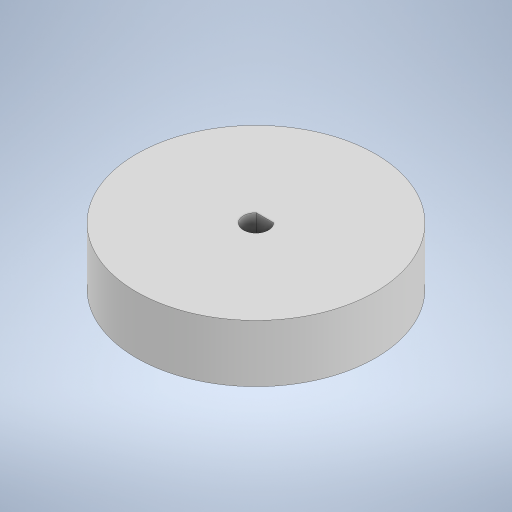
# Autodesk Inventor part: motor_gearMK2
Saved by Autodesk Inventor 2023 (Build 270158000, 158)
## iProperties
Created: 2023-03-07
Part Number: motor_gearMK2
Material: Generic
Document SubType Name: Modeling
Designer: caleb
Density: 1 g/cm^3
Appearance: Default
Author: caleb
Autodesk Inventor part; units mm, degrees
ref_plane "YZ Plane" through (0, 0, 0) normal (1, 0, 0) x (0, 1, 0)
ref_plane "XZ Plane" through (0, 0, 0) normal (0, 1, 0) x (-1, 0, 0)
ref_plane "XY Plane" through (0, 0, 0) normal (0, 0, 1) x (1, 0, 0)
sketch "Sketch1" plane through (0, 0, 0) normal (0, 1, 0) x (-1, 0, 0)
  circle A0 centre (0, 0) radius 25
  circle A1 centre (0, 0) radius 2.625
  line L0 (0, 2.625) -> (0, -1.875)
  line L1 (0, -1.875) -> (1.8371, -1.875)
  line L2 (0, -1.875) -> (-1.8371, -1.875)
  line L3 (27.107, -3.5241) -> (24.4874, -5.0366)
  line L4 (27.0959, 3.6717) -> (24.4538, 5.1971)
  line L5 (27.0959, 3.6717) -> (27.107, -3.5241)
  line L6 (26.1969, 7.8059) -> (24.4189, 5.3588)
  line L7 (23.2599, 14.3752) -> (26.1969, 7.8059)
  line L8 (23.2599, 14.3752) -> (20.2258, 14.6941)
  line L9 (20.7571, 17.7863) -> (20.1282, 14.8276)
  line L10 (15.4021, 22.593) -> (20.7571, 17.7863)
  line L11 (15.4021, 22.593) -> (12.5006, 21.6503)
  line L12 (11.7282, 24.6913) -> (12.3571, 21.7325)
  line L13 (4.8811, 26.9044) -> (11.7282, 24.6913)
  line L14 (4.8811, 26.9044) -> (2.6139, 24.863)
  line L15 (0.6714, 27.3269) -> (2.4493, 24.8797)
  line L16 (-6.4839, 26.5637) -> (0.6714, 27.3269)
  line L17 (-6.4839, 26.5637) -> (-7.7248, 23.7766)
  line L18 (-10.5015, 25.2374) -> (-7.8819, 23.725)
  line L19 (-16.7277, 21.6299) -> (-10.5015, 25.2374)
  line L20 (-16.7277, 21.6299) -> (-16.7277, 18.5791)
  line L21 (-19.8586, 18.7842) -> (-16.8503, 18.468)
  line L22 (-24.0792, 12.9561) -> (-19.8586, 18.7842)
  line L23 (-24.0792, 12.9561) -> (-22.8383, 10.1691)
  line L24 (-25.7819, 9.083) -> (-22.9051, 10.0177)
  line L25 (-27.2672, 2.0421) -> (-25.7819, 9.083)
  line L26 (-27.2672, 2.0421) -> (-25, 0.0007)
  line L27 (-27.2473, -2.1887) -> (-24.9995, -0.1647)
  line L28 (-25.7404, -9.225) -> (-27.2473, -2.1887)
  line L29 (-25.7404, -9.225) -> (-22.8389, -10.1678)
  line L30 (-24.0015, -13.082) -> (-22.7711, -10.3187)
  line L31 (-19.7629, -18.897) -> (-24.0015, -13.082)
  line L32 (-19.7629, -18.897) -> (-16.7288, -18.5781)
  line L33 (-16.6055, -21.7133) -> (-16.6055, -18.6884)
  line L34 (-10.3682, -25.3016) -> (-16.6055, -21.7133)
  line L35 (-10.3682, -25.3016) -> (-7.7261, -23.7762)
  line L36 (-6.3383, -26.5901) -> (-7.5686, -23.8268)
  line L37 (0.8193, -27.3313) -> (-6.3383, -26.5901)
  line L38 (0.8193, -27.3313) -> (2.6125, -24.8631)
  line L39 (5.0249, -26.8693) -> (2.777, -24.8453)
  line L40 (11.8651, -24.6351) -> (5.0249, -26.8693)
  line L41 (11.8651, -24.6351) -> (12.4994, -21.651)
  line L42 (15.5192, -22.5025) -> (12.6424, -21.5678)
  line L43 (20.8593, -17.6793) -> (15.5192, -22.5025)
  line L44 (20.8593, -17.6793) -> (20.225, -14.6952)
  line L45 (23.3301, -14.2449) -> (20.3218, -14.5611)
  line L46 (26.2468, -7.6666) -> (23.3301, -14.2449)
  line L47 (26.2468, -7.6666) -> (24.4535, -5.1985)
  point P0 (20.2258, 14.6941)
  point P1 (24.4189, 5.3588)
  point P2 (12.5006, 21.6503)
  point P3 (20.1282, 14.8276)
  point P4 (2.6139, 24.863)
  point P5 (12.3571, 21.7325)
  point P6 (-7.7248, 23.7766)
  point P7 (2.4493, 24.8797)
  point P8 (-16.7277, 18.5791)
  point P9 (-7.8819, 23.725)
  point P10 (-22.8383, 10.1691)
  point P11 (-16.8503, 18.468)
  point P12 (-25, 0.0007)
  point P13 (-22.9051, 10.0177)
  point P14 (-22.8389, -10.1678)
  point P15 (-24.9995, -0.1647)
  point P16 (-16.7288, -18.5781)
  point P17 (-22.7711, -10.3187)
  point P18 (-7.7261, -23.7762)
  point P19 (-16.6055, -18.6884)
  point P20 (2.6125, -24.8631)
  point P21 (-7.5686, -23.8268)
  point P22 (12.4994, -21.651)
  point P23 (2.777, -24.8453)
  point P24 (20.225, -14.6952)
  point P25 (12.6424, -21.5678)
  point P26 (24.4535, -5.1985)
  point P27 (20.3218, -14.5611)
  dimension "d0" = 50
  dimension "d1" = 5.25
  dimension "d2" = 4.5
  dimension "d24" = 360
  constraints: 96 end point, 3 point on circle, 2 coincident, 1 centre point, 1 horizontal, 1 point on line, 1 vertical, 110 other
  measures "d1" diameter of A1
  measures "d2" distance of L0.start L0.end
extrude "Extrusion2" add sketch "Sketch1" along normal blind 12 contours A0 | A1 L2 L1
body "Solid2"
